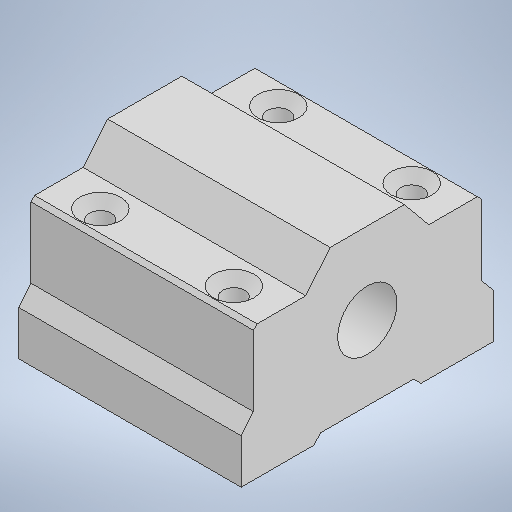
# Autodesk Inventor part: Bearing block
Saved by Autodesk Inventor 2025.2 (Build 292293000, 293)
## iProperties
Created: 2025-01-26
Part Number: Bearing block
Material: Generic
Document SubType Name: Modeling
Designer: caomi
Density: 1 g/cm^3
Appearance: Default
Author: caomi
Autodesk Inventor part; units mm, degrees
ref_plane "YZ Plane" through (0, 0, 0) normal (1, 0, 0) x (0, 1, 0)
ref_plane "XZ Plane" through (0, 0, 0) normal (0, 1, 0) x (-1, 0, 0)
ref_plane "XY Plane" through (0, 0, 0) normal (0, 0, 1) x (1, 0, 0)
sketch "Sketch1" plane through (0, 0, 0) normal (1, 0, 0) x (0, 1, 0)
  line L0 (14.2461, 0) -> (-14.2461, 0) construction
  line L1 (11, 5) -> (11, -5)
  line L2 (11, -5) -> (7, -8.3)
  line L3 (7, -8.3) -> (7, -15.35)
  line L4 (7, -15.35) -> (-3, -15.35)
  line L5 (-3, -15.35) -> (-5, -17)
  line L6 (-5, -17) -> (-11, -17)
  line L7 (-11, 17) -> (-5, 17)
  line L8 (-5, 17) -> (-3, 15.35)
  line L9 (-3, 15.35) -> (7, 15.35)
  line L10 (7, 15.35) -> (7, 8.3)
  line L11 (7, 8.3) -> (11, 5)
  line L12 (-11, -17) -> (-11, -7.25)
  line L13 (-11, -7.25) -> (-10, -6.25)
  line L14 (-10, -6.25) -> (-10, 6.25)
  line L15 (-10, 6.25) -> (-11, 7.25)
  line L16 (-11, 7.25) -> (-11, 17)
  circle A0 centre (0, 0) radius 4
  point P0 (-11, -12.125)
  dimension "d2" = 45
  dimension "d3" = 22
  dimension "d4" = 34
  dimension "d5" = 6
  dimension "d6" = 8
  dimension "d7" = 11
  dimension "d8" = 8
  dimension "d9" = 18
  dimension "d10" = 16.6
  dimension "d11" = 12.5
  dimension "d12" = 1
  dimension "d13" = 10
  constraints: 34 end point, 5 parallel, 3 midpoint, 2 perpendicular, 2 vertical, 1 centre point, 1 collinear, 1 horizontal, 1 point on line, 7 other
  measures "d2" angle of L12 L13
  measures "d3" distance from line of point (-11, -12.125) L1
  measures "d4" distance between parallel lines of L7 L6
  measures "d5" distance of L5.end L6.end
  measures "d6" distance from line of L12 L4.end
  measures "d7" distance from line of A0.centre L16
  measures "d8" diameter of A0
  measures "d9" distance between parallel lines of L12 L3
  measures "d10" distance of L2.end L10.end
  measures "d11" distance of L13.end L14.end
  measures "d12" distance between parallel lines of L14 L12
  measures "d13" distance of L1.start L1.end
extrude "Extrusion1" add sketch "Sketch1" along normal mid plane 30
sketch "Sketch2" plane through (-15, 7, 15.35) normal (0, 1, 0) x (1, 0, 0)
  line L0 (-4.3659, 15.35) -> (34.0137, 15.35) construction
  line L1 (0, 10.35) -> (0, 20.35) projected
  line L2 (0, 10.35) -> (30, 10.35) projected
  line L3 (15, 2.4961) -> (15, 28.0168) construction
  point P0 (15, 15.35)
  point P1 (6, 3.35)
  point P2 (6, 27.35)
  point P3 (24, 27.35)
  point P4 (24, 3.35)
  point P5 (0, 15.35)
  point P6 (15, 10.35)
  dimension "d16" = 24
  dimension "d17" = 18
  constraints: 4 end point, 2 horizontal alignment, 2 midpoint, 2 point on line, 2 symmetric about line, 2 vertical alignment, 1 horizontal, 1 vertical
  measures "d16" distance of point (6, 3.35) point (6, 27.35)
  measures "d17" distance of point (24, 3.35) point (6, 3.35)
hole "Hole1" at (-9, 7, 12) at (-9, 7, -12) at (9, 7, -12) at (9, 7, 12) direction (0, -1, 0) diameter 3 depth 8 countersink diameter 5.5 countersink angle 90
sketch "Sketch3" plane through (-15, -11, 7.25) normal (0, -1, 0) x (1, 0, 0)
  point P0 (15, -7.25)
  point P1 (6, 4.75)
  point P2 (24, 4.75)
  point P3 (6, -19.25)
  point P4 (24, -19.25)
hole "Hole2" at (-9, -11, 12) at (9, -11, 12) at (-9, -11, -12) at (9, -11, -12) direction (0, 1, 0) diameter 3 end through all countersink diameter 5.5 countersink angle 90
chamfer "Chamfer1" distance 0.5 angle 45 2 edges at (0, 7, 15.35) (0, 7, -15.35)
body "Solid1"
